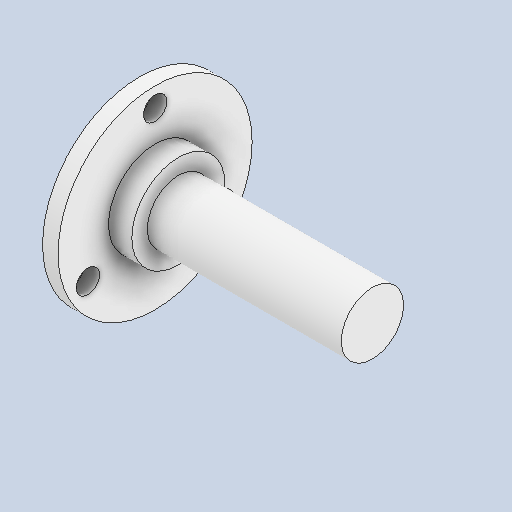
# Autodesk Inventor part: belt_axis
Saved by Autodesk Inventor 2025.3 (Build 293356030, 356C)
## iProperties
Created: 2025-09-21
Part Number: belt_axis
Material: PLA+ filament
Document SubType Name: Modeling
Designer: MSI
Mass: 3.11838 g
Surface Area: 18.9438 cm^2
Volume: 2.53527 cm^3
Density: 1.23 g/cm^3
Appearance: 일반
Author: MSI
Autodesk Inventor part; units mm, degrees
ref_plane "YZ Plane" through (0, 0, 0) normal (1, 0, 0) x (0, 1, 0)
ref_plane "XZ Plane" through (0, 0, 0) normal (0, 1, 0) x (-1, 0, 0)
ref_plane "XY Plane" through (0, 0, 0) normal (0, 0, 1) x (1, 0, 0)
sketch "스케치1" plane through (0, 0, 0) normal (0, 0, 1) x (1, 0, 0)
  line L0 (-30, 0) -> (30, 0)
  line L1 (2, 12.5) -> (2, 6)
  line L2 (2, 6) -> (5, 6)
  line L3 (5, 6) -> (5, 4)
  line L4 (5, 4) -> (30, 4)
  line L5 (30, 4) -> (30, 0)
  line L6 (2, 12.5) -> (0, 12.5)
  line L7 (0, 12.5) -> (0, 0)
  dimension "d1" = 12
  dimension "d2" = 8
  dimension "d4" = 3
  dimension "d5" = 25
  dimension "d7" = 25
  dimension "d8" = 2
  constraints: 17 end point, 5 perpendicular, 2 horizontal, 1 coincident, 1 midpoint
  measures "d1" diameter of L2 L0
  measures "d2" diameter of L4 L0
  measures "d4" distance of L1.end L2.end
  measures "d5" distance of L3.end L4.end
  measures "d7" diameter of L6 L0
  measures "d8" distance of L1.start L6.end
revolve "회전1" add sketch "스케치1" angle 360 about axis through (-30, 0, 0) along (1, 0, 0)
sketch "스케치2" plane through (0, 0, 0) normal (-1, 0, 0) x (0, 0, 1)
  line L0 (0, 0) -> (0, 10) construction
  dimension "d9" = 10
  constraints: 2 end point, 1 vertical
  measures "d9" distance of L0.start L0.end
hole "구멍1" at (0, 10, 0) direction (1, 0, 0) diameter 3 depth 2
pattern_circular "원형 패턴1" count 3 over 360 about axis through (1, 0, 0) along (1, 0, 0) of "구멍1"
